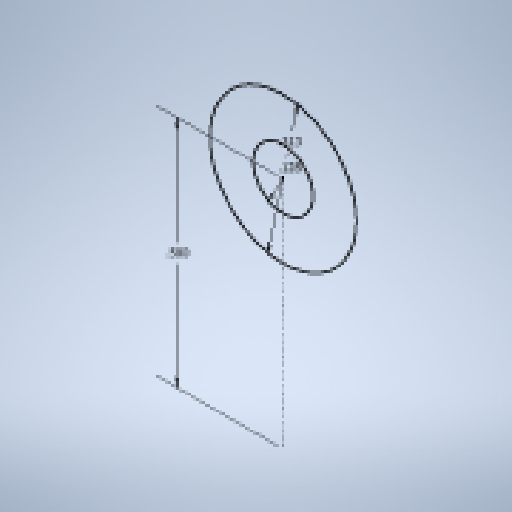
# Autodesk Inventor part: Hinge
Saved by Autodesk Inventor 2023.4 (Build 274418000, 418)
## iProperties
Created: 2024-07-02
Part Number: Hinge
Material: Generic
Document SubType Name: Modeling
Designer: Nathan Cai
Density: 1 g/cm^3
Appearance: Default
Author: Nathan Cai
Autodesk Inventor part; units mm, degrees
ref_plane "YZ Plane" through (0, 0, 0) normal (1, 0, 0) x (0, 1, 0)
ref_plane "XZ Plane" through (0, 0, 0) normal (0, 1, 0) x (-1, 0, 0)
ref_plane "XY Plane" through (0, 0, 0) normal (0, 0, 1) x (1, 0, 0)
sketch "Sketch1" plane through (0, 0, 0) normal (0, 0, 1) x (1, 0, 0)
  line L0 (0, 0) -> (0, 12.7) construction
  circle A0 centre (0, 12.7) radius 1.625
  circle A1 centre (0, 12.7) radius 3.9688
  line L1 (-1.5875, -9.0626) -> (1.5875, -9.0626) construction
  line L2 (1.5875, -9.0626) -> (1.5875, 9.0626)
  line L3 (1.5875, 9.0626) -> (-1.5875, 9.0626) construction
  line L4 (-1.5875, 9.0626) -> (-1.5875, -9.0626)
  line L5 (-1.5875, -9.0626) -> (1.5875, 9.0626) construction
  line L6 (1.5875, -9.0626) -> (-1.5875, 9.0626) construction
  circle A2 centre (0, -12.7) radius 1.625
  circle A3 centre (0, -12.7) radius 3.9688
  line L7 (-1.5875, -9.0626) -> (1.5875, -9.0626) construction
  line L8 (-2.3813, -4.7625) -> (-0.7937, -4.7625)
  line L9 (-0.7937, -4.7625) -> (-0.7937, 4.7625)
  line L10 (-0.7937, 4.7625) -> (-2.3813, 4.7625)
  line L11 (-2.3813, 4.7625) -> (-2.3813, -4.7625) construction
  line L12 (-2.3813, -4.7625) -> (-0.7937, 4.7625) construction
  line L13 (-0.7937, -4.7625) -> (-2.3813, 4.7625) construction
  line L14 (0.7937, -4.7625) -> (2.3813, -4.7625)
  line L15 (2.3813, -4.7625) -> (2.3813, 4.7625)
  line L16 (2.3813, 4.7625) -> (0.7937, 4.7625)
  line L17 (0.7937, 4.7625) -> (0.7937, -4.7625) construction
  line L18 (0.7937, -4.7625) -> (2.3813, 4.7625) construction
  line L19 (2.3813, -4.7625) -> (0.7937, 4.7625) construction
  point P0 (-1.5875, 0)
  point P1 (1.5875, 0)
  point P2 (-1.5875, 4.7625)
  point P3 (-1.5875, -4.7625)
  point P4 (1.5875, -4.7625)
  point P5 (1.5875, 4.7625)
  dimension "d2" = 7.9375
  dimension "d0" = 12.7
  dimension "d1" = 3.25
  dimension "d3" = 3.175
  dimension "d6" = 360
  dimension "d8" = 1.5875
  dimension "d9" = 9.525
  dimension "d10" = 1.5875
  dimension "d11" = 9.525
  constraints: 40 end point, 8 midpoint, 6 parallel, 4 coincident, 3 horizontal, 3 perpendicular, 2 centre point, 1 vertical, 23 other
  measures "d0" distance of L0.start L0.end
  measures "d1" diameter of A0
  measures "d3" distance of L3.end L2.end
  measures "d8" distance of L10.end L9.end
  measures "d9" distance of L9.end L8.end
  measures "d10" distance of L16.end L15.end
  measures "d11" distance of L15.end L14.end
extrude "Extrusion1" add sketch "Sketch1" along normal blind 12.7 contours A1 | A1 L2 A3 L4 L8 L9 L10 | L16 L15 L14 L2 | A3
chamfer "Chamfer1" distance 0.7937 angle 45 4 edges at (-1.5875, 4.7625, 6.35) (1.5875, 4.7625, 6.35) (1.5875, -4.7625, 6.35) (-1.5875, -4.7625, 6.35)
fillet "Fillet1" radius 3.175 4 edges at (1.5875, 9.0626, 6.35) (-1.5875, 9.0626, 6.35) (1.5875, -9.0626, 6.35) (-1.5875, -9.0626, 6.35)
body "Solid1"
